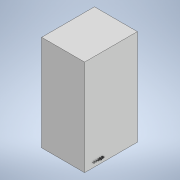
# Autodesk Inventor part: part
Saved by Autodesk Inventor 2021.2 (Build 252289000, 289)
## iProperties
Created: 2021-03-05
Part Number: part
Material: Generic
Document SubType Name: Modeling
Designer: nagyad
Density: 1 g/cm^3
Appearance: Default
Author: nagyad
Autodesk Inventor part; units mm, degrees
note: some values were not read from the file. Chosen so that the rebuilt part matches the saved one: direction of "Emboss1".
ref_plane "YZ Plane" through (0, 0, 0) normal (1, 0, 0) x (0, 1, 0)
ref_plane "XZ Plane" through (0, 0, 0) normal (0, 1, 0) x (-1, 0, 0)
ref_plane "XY Plane" through (0, 0, 0) normal (0, 0, 1) x (1, 0, 0)
sketch "Sketch1" plane through (0, 0, 0) normal (0, 1, 0) x (-1, 0, 0)
  line L0 (0, 0) -> (11.3921, 0)
  line L1 (11.3921, 0) -> (11.3921, -13.9984)
  line L2 (11.3921, -13.9984) -> (0, -13.9984)
  line L3 (0, -13.9984) -> (0, 0)
  constraints: 8 end point, 2 parallel, 1 horizontal, 1 perpendicular
extrude "Extrusion1" add sketch "Sketch1" along normal blind 25.4
sketch "Sketch2" plane through (0, 0, 0) normal (1, 0, 0) x (0, 0, -1)
  line L0 (2.0058, 1.5555) -> (10.2338, 1.5555) construction
  line L1 (10.2338, 1.5555) -> (10.2338, 0.614) construction
  line L2 (10.2338, 0.614) -> (2.0058, 0.614) construction
  line L3 (2.0058, 0.614) -> (2.0058, 1.5555) construction
  line L4 (2.441, 1.071) -> (2.0746, 1.246)
  line L5 (2.0746, 1.246) -> (2.0746, 1.2867)
  line L6 (2.0746, 1.2867) -> (2.441, 1.4617)
  line L7 (2.441, 1.4617) -> (2.441, 1.4012)
  line L8 (2.441, 1.4012) -> (2.1569, 1.2665)
  line L9 (2.1569, 1.2665) -> (2.441, 1.1315)
  line L10 (2.441, 1.1315) -> (2.441, 1.071)
  line L11 (2.9494, 1.071) -> (2.583, 1.246)
  line L12 (2.583, 1.246) -> (2.583, 1.2867)
  line L13 (2.583, 1.2867) -> (2.9494, 1.4617)
  line L14 (2.9494, 1.4617) -> (2.9494, 1.4012)
  line L15 (2.9494, 1.4012) -> (2.6653, 1.2665)
  line L16 (2.6653, 1.2665) -> (2.9494, 1.1315)
  line L17 (2.9494, 1.1315) -> (2.9494, 1.071)
  spline S0 degree 2 poles (3.6006, 1.2349) (3.6006, 1.1385) (3.508, 1.0335) (3.4306, 1.0335) knots 0 0 0 1 2 2 2
  spline S1 degree 2 poles (3.4306, 1.0335) (3.3512, 1.0335) (3.2602, 1.1418) (3.2602, 1.2349) knots 0 0 0 1 2 2 2
  spline S2 degree 2 poles (3.2602, 1.2349) (3.2602, 1.3304) (3.354, 1.4362) (3.4306, 1.4362) knots 0 0 0 1 2 2 2
  spline S3 degree 2 poles (3.4306, 1.4362) (3.508, 1.4362) (3.6006, 1.3308) (3.6006, 1.2349) knots 0 0 0 1 2 2 2
  spline S4 degree 2 poles (3.5344, 1.2349) (3.5344, 1.309) (3.4804, 1.381) (3.4306, 1.381) knots 0 0 0 1 2 2 2
  spline S5 degree 2 poles (3.4306, 1.381) (3.3808, 1.381) (3.3265, 1.309) (3.3265, 1.2349) knots 0 0 0 1 2 2 2
  spline S6 degree 2 poles (3.3265, 1.2349) (3.3265, 1.1628) (3.3808, 1.0887) (3.4306, 1.0887) knots 0 0 0 1 2 2 2
  spline S7 degree 2 poles (3.4306, 1.0887) (3.48, 1.0887) (3.5344, 1.1616) (3.5344, 1.2349) knots 0 0 0 1 2 2 2
  line L18 (3.8686, 1.3567) -> (3.8653, 1.3567)
  spline S8 degree 2 poles (3.8653, 1.3567) (3.8579, 1.3588) (3.8419, 1.3596) (3.8308, 1.3596) knots 0 0 0 1 2 2 2
  spline S9 degree 2 poles (3.8308, 1.3596) (3.8048, 1.3596) (3.7538, 1.3369) (3.7307, 1.3147) knots 0 0 0 1 2 2 2
  line L19 (3.7307, 1.3147) -> (3.7307, 1.0442)
  line L20 (3.7307, 1.0442) -> (3.6665, 1.0442)
  line L21 (3.6665, 1.0442) -> (3.6665, 1.4255)
  line L22 (3.6665, 1.4255) -> (3.7307, 1.4255)
  line L23 (3.7307, 1.4255) -> (3.7307, 1.3686)
  spline S10 degree 2 poles (3.7307, 1.3686) (3.7657, 1.3999) (3.818, 1.4255) (3.8427, 1.4255) knots 0 0 0 1 2 2 2
  spline S11 degree 2 poles (3.8427, 1.4255) (3.8526, 1.4255) (3.8625, 1.4246) (3.8686, 1.4234) knots 0 0 0 1 2 2 2
  line L24 (3.8686, 1.4234) -> (3.8686, 1.3567)
  line L25 (3.9839, 1.0442) -> (3.9197, 1.0442)
  line L26 (3.9197, 1.0442) -> (3.9197, 1.4255)
  line L27 (3.9197, 1.4255) -> (3.9839, 1.4255)
  line L28 (3.9839, 1.4255) -> (3.9839, 1.0442)
  line L29 (3.9884, 1.4889) -> (3.9156, 1.4889)
  line L30 (3.9156, 1.4889) -> (3.9156, 1.5555)
  line L31 (3.9156, 1.5555) -> (3.9884, 1.5555)
  line L32 (3.9884, 1.5555) -> (3.9884, 1.4889)
  spline S12 degree 2 poles (4.0918, 0.9833) (4.0983, 0.9804) (4.1235, 0.9714) (4.1395, 0.9677) knots 0 0 0 1 2 2 2
  spline S13 degree 2 poles (4.1395, 0.9677) (4.1572, 0.9631) (4.1873, 0.9578) (4.205, 0.9578) knots 0 0 0 1 2 2 2
  spline S14 degree 2 poles (4.205, 0.9578) (4.2346, 0.9578) (4.2758, 0.9734) (4.2873, 0.9874) knots 0 0 0 1 2 2 2
  spline S15 degree 2 poles (4.2873, 0.9874) (4.2984, 1.0014) (4.3071, 1.0381) (4.3071, 1.0615) knots 0 0 0 1 2 2 2
  line L33 (4.3071, 1.0615) -> (4.3071, 1.0949)
  spline S16 degree 2 poles (4.3071, 1.0949) (4.2811, 1.0722) (4.2313, 1.0508) (4.1939, 1.0508) knots 0 0 0 1 2 2 2
  spline S17 degree 2 poles (4.1939, 1.0508) (4.1288, 1.0508) (4.0518, 1.1476) (4.0518, 1.2386) knots 0 0 0 1 2 2 2
  spline S18 degree 2 poles (4.0518, 1.2386) (4.0518, 1.2859) (4.0786, 1.3592) (4.1008, 1.3851) knots 0 0 0 1 2 2 2
  spline S19 degree 2 poles (4.1008, 1.3851) (4.1222, 1.4094) (4.1811, 1.4362) (4.2124, 1.4362) knots 0 0 0 1 2 2 2
  spline S20 degree 2 poles (4.2124, 1.4362) (4.242, 1.4362) (4.2852, 1.4222) (4.3071, 1.4094) knots 0 0 0 1 2 2 2
  line L34 (4.3071, 1.4094) -> (4.3108, 1.4255)
  line L35 (4.3108, 1.4255) -> (4.3713, 1.4255)
  line L36 (4.3713, 1.4255) -> (4.3713, 1.0879)
  spline S21 degree 2 poles (4.3713, 1.0879) (4.3713, 0.9907) (4.2869, 0.9002) (4.2, 0.9002) knots 0 0 0 1 2 2 2
  spline S22 degree 2 poles (4.2, 0.9002) (4.172, 0.9002) (4.1136, 0.9092) (4.0885, 0.9166) knots 0 0 0 1 2 2 2
  line L37 (4.0885, 0.9166) -> (4.0885, 0.9833)
  line L38 (4.0885, 0.9833) -> (4.0918, 0.9833)
  line L39 (4.3071, 1.1476) -> (4.3071, 1.3571)
  spline S23 degree 2 poles (4.3071, 1.3571) (4.2832, 1.3686) (4.2428, 1.3785) (4.2227, 1.3785) knots 0 0 0 1 2 2 2
  spline S24 degree 2 poles (4.2227, 1.3785) (4.1741, 1.3785) (4.1181, 1.3069) (4.1181, 1.2398) knots 0 0 0 1 2 2 2
  spline S25 degree 2 poles (4.1181, 1.2398) (4.1181, 1.1764) (4.1605, 1.1101) (4.2083, 1.1101) knots 0 0 0 1 2 2 2
  spline S26 degree 2 poles (4.2083, 1.1101) (4.2334, 1.1101) (4.2861, 1.1299) (4.3071, 1.1476) knots 0 0 0 1 2 2 2
  line L40 (4.5298, 1.0442) -> (4.4656, 1.0442)
  line L41 (4.4656, 1.0442) -> (4.4656, 1.4255)
  line L42 (4.4656, 1.4255) -> (4.5298, 1.4255)
  line L43 (4.5298, 1.4255) -> (4.5298, 1.0442)
  line L44 (4.5343, 1.4889) -> (4.4614, 1.4889)
  line L45 (4.4614, 1.4889) -> (4.4614, 1.5555)
  line L46 (4.4614, 1.5555) -> (4.5343, 1.5555)
  line L47 (4.5343, 1.5555) -> (4.5343, 1.4889)
  line L48 (4.9233, 1.0442) -> (4.8591, 1.0442)
  line L49 (4.8591, 1.0442) -> (4.8591, 1.2616)
  spline S27 degree 2 poles (4.8591, 1.2616) (4.8591, 1.288) (4.8542, 1.3332) (4.8468, 1.3468) knots 0 0 0 1 2 2 2
  spline S28 degree 2 poles (4.8468, 1.3468) (4.8389, 1.3612) (4.8109, 1.3752) (4.7871, 1.3752) knots 0 0 0 1 2 2 2
  spline S29 degree 2 poles (4.7871, 1.3752) (4.7632, 1.3752) (4.7126, 1.3497) (4.6883, 1.3291) knots 0 0 0 1 2 2 2
  line L50 (4.6883, 1.3291) -> (4.6883, 1.0442)
  line L51 (4.6883, 1.0442) -> (4.624, 1.0442)
  line L52 (4.624, 1.0442) -> (4.624, 1.4255)
  line L53 (4.624, 1.4255) -> (4.6883, 1.4255)
  line L54 (4.6883, 1.4255) -> (4.6883, 1.3831)
  spline S30 degree 2 poles (4.6883, 1.3831) (4.7171, 1.409) (4.7727, 1.4362) (4.8039, 1.4362) knots 0 0 0 1 2 2 2
  spline S31 degree 2 poles (4.8039, 1.4362) (4.8599, 1.4362) (4.9233, 1.3621) (4.9233, 1.2917) knots 0 0 0 1 2 2 2
  line L55 (4.9233, 1.2917) -> (4.9233, 1.0442)
  point P0 (0, 0)
  constraints: 2 other
emboss "Emboss1" sketch "Sketch2" operation add depth 0.254 direction (-1, 0, 0)
body "Solid1"
